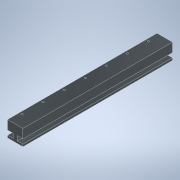
# Autodesk Inventor part: Балка
Saved by Autodesk Inventor 2021 (Build 250183000, 183)
## iProperties
Created: 2020-12-05
Part Number: Балка
Material: Чугун, серый
Document SubType Name: Modeling
Designer: Тимоха
Mass: 11560.1 g
Surface Area: 1692 cm^2
Volume: 1616.8 cm^3
Density: 7.15 g/cm^3
Appearance: Чугун серый
Author: Тимоха
Autodesk Inventor part; units mm, degrees
ref_plane "YZ Plane" through (0, 0, 0) normal (1, 0, 0) x (0, 1, 0)
ref_plane "XZ Plane" through (0, 0, 0) normal (0, 1, 0) x (-1, 0, 0)
ref_plane "XY Plane" through (0, 0, 0) normal (0, 0, 1) x (1, 0, 0)
sketch "Эскиз1" plane through (0, 0, 0) normal (0, 0, 1) x (1, 0, 0)
  line L0 (0, 0) -> (68, 0)
  line L1 (68, 0) -> (68, -70)
  line L2 (68, -70) -> (0, -70)
  line L3 (0, -70) -> (0, 0)
  line L4 (0, 0) -> (0, -40)
  line L5 (0, -40) -> (25, -40)
  line L6 (25, -40) -> (25, -60)
  line L7 (25, -60) -> (0, -60)
  line L8 (34, 0) -> (34, -70)
  line L9 (68, -40) -> (43, -40)
  line L10 (43, -40) -> (43, -60)
  line L11 (43, -60) -> (68, -60)
  dimension "d0" = 68
  dimension "d1" = 70
  dimension "d2" = 40
  dimension "d3" = 25
  dimension "d4" = 20
  constraints: 24 end point, 4 perpendicular, 4 symmetric about line, 2 midpoint, 2 parallel, 2 point on line, 1 horizontal
  measures "d0" distance of L1.end L2.end
  measures "d1" distance of L0.end L1.end
  measures "d2" distance of L0.start L4.end
  measures "d3" distance of L4.end L5.end
  measures "d4" distance of L5.end L6.end
extrude "Выдавливание1" add sketch "Эскиз1" along normal blind 660 contours L0 L8 L2 L3 L7 L6 L5 | L0 L1 L9 L10 L11 L2 L8
sketch "Эскиз2" plane through (0, 0, 0) normal (0, 1, 0) x (1, 0, 0)
  circle A0 centre (12, 10) radius 4 projected
  line L0 (12, 10) -> (12, -50)
  point P0 (0, 0)
  dimension "d7" = 60
  constraints: 2 end point, 1 vertical
  measures "d7" distance of L0.start L0.end
hole "Отверстие1" at (12, 0, 50) direction (0, -1, 0) diameter 6 depth 17 tip angle 118 counterbore diameter 8 counterbore depth 12
pattern_linear "Прямоуг.массив1" count 7 spacing 93 along (0, 0, 1) of "Отверстие1"
ref_plane "РабПлоскость1" through (34, -40, 0) normal (1, 0, 0) x (0, 0, -1)
mirror "Зеркальное отражение1" about plane through (34, -40, 0) normal (1, 0, 0) of "Отверстие1", "Прямоуг.массив1"
